Autodesk Inventor part; units mm, degrees
(part 3 of 3)
sketch "Sketch11" plane through (0, 0, 6.35) normal (0, 0, 1) x (1, 0, 0)
  line L0 (-44.1315, -133.8713) -> (-53.8141, -133.1794)
  arc A0 (-51.8719, -136.3964) -> (-74.636, -135.0027) centre (-63.5956, -141.2796) ccw projected
  line L1 (-36.4798, -134.4181) -> (-44.1315, -133.8713) projected
  arc A1 (-79.0465, -94.081) -> (-76.0542, -98.0205) centre (-69.1827, -89.6949) ccw projected
  line L2 (-76.0542, -98.0205) -> (-35.3561, -131.6103) projected
  arc A2 (-36.4798, -134.4181) -> (-35.3561, -131.6103) centre (-36.3666, -132.8347) ccw projected
  line L3 (-36.4798, -134.4181) -> (-44.1315, -133.8713) projected
  arc A3 (-44.1315, -133.8713) -> (-51.8719, -136.3964) centre (-44.901, -144.6389) ccw projected
  arc A4 (-51.8719, -136.3964) -> (-74.636, -135.0027) centre (-63.5956, -141.2796) ccw projected
  arc A5 (-85.5845, -139.4581) -> (-93.4453, -121.7039) centre (-97.0428, -133.914) ccw projected
  line L4 (-93.4453, -121.7039) -> (-88.3661, -96.7346) projected
  arc A6 (-88.3661, -96.7346) -> (-79.0465, -94.081) centre (-86.9165, -84.1335) ccw projected
  arc A7 (-88.6509, -203.8227) -> (-105.452, -206.2132) centre (-93.2079, -232.032) ccw projected
  arc A8 (-109.9237, -202.7115) -> (-105.452, -206.2132) centre (-106.8124, -203.3444) ccw projected
  line L5 (-109.9237, -202.7115) -> (-109.1471, -198.8936) projected
  arc A9 (-106.259, -196.3593) -> (-109.1471, -198.8936) centre (-106.0358, -199.5265) ccw projected
  arc A10 (-106.259, -196.3593) -> (-98.2138, -192.7133) centre (-107.1516, -183.6907) ccw projected
  arc A11 (-94.937, -191.9699) -> (-98.2138, -192.7133) centre (-95.9794, -194.9689) ccw projected
  line L6 (-94.937, -191.9699) -> (-86.0461, -195.0603) projected
  arc A12 (-84.1423, -199.2428) -> (-86.0461, -195.0603) centre (-87.0885, -198.0593) ccw projected
  line L7 (-84.1423, -199.2428) -> (-85.1984, -201.8718) projected
  arc A13 (-88.6509, -203.8227) -> (-85.1984, -201.8718) centre (-88.1445, -200.6883) ccw projected
  arc A14 (-28.8339, -52.5673) -> (-24.5425, -50.8749) centre (-27.4887, -49.6914) ccw projected
  line L8 (-28.8339, -52.5673) -> (-62.2456, -36.9383) projected
  arc A15 (-64.0748, -34.1198) -> (-62.2456, -36.9383) centre (-60.9004, -34.0624) ccw projected
  arc A16 (-64.0748, -34.1198) -> (-69.5395, -23.9103) centre (-76.7728, -34.3492) ccw projected
  arc A17 (-70.5556, -19.8503) -> (-69.5395, -23.9103) centre (-67.7312, -21.3006) ccw projected
  arc A18 (-64.7921, -10.8231) -> (-70.5556, -19.8503) centre (-19.7163, -45.9555) ccw projected
  line L9 (-64.7921, -10.8231) -> (-52.5861, 4.8375) projected
  arc A19 (-46.9122, 2.703) -> (-52.5861, 4.8375) centre (-50.0819, 2.8857) ccw projected
  arc A20 (-46.9122, 2.703) -> (-23.4164, -40.7398) centre (0, 0) ccw projected
  arc A21 (-22.0524, -44.676) -> (-23.4164, -40.7398) centre (-24.9986, -43.4925) ccw projected
  line L10 (-22.0524, -44.676) -> (-24.5425, -50.8749) projected
  arc A22 (-88.5389, -146.9454) -> (-92.3649, -145.7242) centre (-91.1997, -148.6777) ccw projected
  line L11 (-88.5389, -146.9454) -> (-60.6625, -189.7642) projected
  arc A23 (-61.0938, -193.7571) -> (-60.6625, -189.7642) centre (-63.3233, -191.4965) ccw projected
  arc A24 (-61.0938, -193.7571) -> (-61.1139, -193.7769) centre (-52.1761, -202.7994) ccw projected
  arc A25 (-64.3907, -194.5202) -> (-61.1139, -193.7769) centre (-63.3483, -191.5212) ccw projected
  line L12 (-64.3907, -194.5202) -> (-92.4352, -184.7723) projected
  arc A26 (-94.5445, -182.1568) -> (-92.4352, -184.7723) centre (-91.3928, -181.7733) ccw projected
  arc A27 (-94.5445, -182.1568) -> (-101.3806, -172.3776) centre (-107.1516, -183.6907) ccw projected
  arc A28 (-103.0492, -168.9165) -> (-101.3806, -172.3776) centre (-99.9379, -169.5493) ccw projected
  line L13 (-103.0492, -168.9165) -> (-99.0208, -149.1131) projected
  arc A29 (-96.1327, -146.5788) -> (-99.0208, -149.1131) centre (-95.9095, -149.746) ccw projected
  arc A30 (-96.1327, -146.5788) -> (-92.3649, -145.7242) centre (-97.0253, -133.9102) ccw projected
  arc A31 (-17.7613, -54.4362) -> (-16.1603, -58.4956) centre (-14.8151, -55.6197) ccw projected
  line L14 (-17.7613, -54.4362) -> (-14.9815, -47.5164) projected
  arc A32 (-11.2736, -45.6176) -> (-14.9815, -47.5164) centre (-12.0354, -48.6999) ccw projected
  arc A33 (-11.2736, -45.6176) -> (22.335, -41.3425) centre (0, 0) ccw projected
  arc A34 (26.6735, -45.5766) -> (22.335, -41.3425) centre (23.8442, -44.136) ccw projected
  line L15 (26.6735, -45.5766) -> (18.348, -61.9272) projected
  arc A35 (14.8879, -63.5983) -> (18.348, -61.9272) centre (15.5186, -60.4865) ccw projected
  arc A36 (14.8879, -63.5983) -> (4.4026, -66.1514) centre (12.3652, -76.0452) ccw projected
  arc A37 (1.0666, -66.5539) -> (4.4026, -66.1514) centre (2.4119, -63.6779) ccw projected
  line L16 (1.0666, -66.5539) -> (-16.1603, -58.4956) projected
  arc A38 (-75.9857, -77.6344) -> (-81.1281, -72.8166) centre (-86.899, -84.1297) ccw projected
  arc A39 (-82.7967, -69.3554) -> (-81.1281, -72.8166) centre (-79.6854, -69.9883) ccw projected
  line L17 (-82.7967, -69.3554) -> (-78.7683, -49.5521) projected
  arc A40 (-75.8802, -47.0178) -> (-78.7683, -49.5521) centre (-75.657, -50.185) ccw projected
  arc A41 (-75.8802, -47.0178) -> (-68.8102, -44.243) centre (-76.7728, -34.3492) ccw projected
  arc A42 (-65.4743, -43.8405) -> (-68.8102, -44.243) centre (-66.8195, -46.7164) ccw projected
  line L18 (-65.4743, -43.8405) -> (-13.0907, -68.3439) projected
  arc A43 (-14.1782, -74.3844) -> (-13.0907, -68.3439) centre (-14.436, -71.2199) ccw projected
  line L19 (-14.1782, -74.3844) -> (-72.9996, -79.1751) projected
  arc A44 (-75.9857, -77.6344) -> (-72.9996, -79.1751) centre (-73.2574, -76.0105) ccw projected
  arc A45 (1.4518, -82.5405) -> (3.7832, -85.4068) centre (12.3652, -76.0452) ccw projected
  arc A46 (4.4671, -89.1879) -> (3.7832, -85.4068) centre (1.6378, -87.7473) ccw projected
  line L20 (4.4671, -89.1879) -> (-13.923, -125.3043) projected
  arc A47 (-17.3829, -126.9753) -> (-13.923, -125.3043) centre (-16.7523, -123.8636) ccw projected
  arc A48 (-17.3829, -126.9753) -> (-25.1442, -127.8531) centre (-19.9055, -139.4223) ccw projected
  arc A49 (-28.4749, -127.4095) -> (-25.1442, -127.8531) centre (-26.4539, -124.9608) ccw projected
  line L21 (-28.4749, -127.4095) -> (-71.2037, -92.1436) projected
  arc A50 (-69.4404, -86.5304) -> (-71.2037, -92.1436) centre (-69.1827, -89.6949) ccw projected
  line L22 (-69.4404, -86.5304) -> (-1.5342, -80.9998) projected
  arc A51 (1.4518, -82.5405) -> (-1.5342, -80.9998) centre (-1.2765, -84.1643) ccw projected
  arc A52 (-64.7831, -204.3333) -> (-60.7584, -212.1608) centre (-52.1761, -202.7994) ccw projected
  arc A53 (-60.0746, -215.9418) -> (-60.7584, -212.1608) centre (-62.9039, -214.5011) ccw projected
  line L23 (-60.0746, -215.9418) -> (-61.8773, -219.482) projected
  arc A54 (-67.5567, -219.4404) -> (-61.8773, -219.482) centre (-64.7066, -218.0413) ccw projected
  arc A55 (-67.5567, -219.4404) -> (-76.984, -208.5093) centre (-93.2079, -232.032) ccw projected
  arc A56 (-78.1275, -204.7122) -> (-76.984, -208.5093) centre (-75.1814, -205.8957) ccw projected
  line L24 (-78.1275, -204.7122) -> (-76.8242, -201.4676) projected
  arc A57 (-72.8356, -199.6521) -> (-76.8242, -201.4676) centre (-73.878, -202.6511) ccw projected
  line L25 (-72.8356, -199.6521) -> (-66.8925, -201.7178) projected
  arc A58 (-64.7831, -204.3333) -> (-66.8925, -201.7178) centre (-67.9349, -204.7168) ccw projected
  circle A59 centre (-19.9058, -139.422) radius 5.588 projected
  circle A60 centre (-107.169, -183.6945) radius 5.588 projected
  circle A61 centre (-86.9165, -84.1335) radius 5.588 projected
  circle A62 centre (-56.5448, -157.7983) radius 6.731 projected
  line L26 (-98.521, -236.7409) -> (-93.7871, -224.9561) projected
  arc A63 (-87.8947, -227.3231) -> (-93.7871, -224.9561) centre (-90.8409, -226.1396) ccw projected
  line L27 (-87.8947, -227.3231) -> (-92.6287, -239.1078) projected
  arc A64 (-98.521, -236.7409) -> (-92.6287, -239.1078) centre (-95.5749, -237.9244) ccw projected
  circle A65 centre (0, 0) radius 13.4938 projected
  arc A66 (56.5866, -28.8133) -> (-50.0843, 39.0361) centre (0, 0) ccw projected
  line L28 (-50.0843, 39.0361) -> (-79.8174, 0.8878) projected
  arc A67 (-79.8174, 0.8878) -> (-94.387, -30.7661) centre (-19.7163, -45.9555) ccw projected
  line L29 (-94.387, -30.7661) -> (-133.6545, -223.8044) projected
  arc A68 (-133.6545, -223.8044) -> (-56.4266, -250.7606) centre (-93.2079, -232.032) ccw projected
  line L30 (-56.4266, -250.7606) -> (56.5866, -28.8133) projected
  circle A69 centre (-63.5956, -141.2796) radius 6.731 projected
  arc A70 (-11.6072, -28.8689) -> (-9.2419, -22.976) centre (-10.4066, -25.9296) ccw projected
  arc A71 (-9.2419, -22.976) -> (-11.6072, -28.8689) centre (-10.4425, -25.9152) ccw projected
  arc A72 (26.3454, 16.5542) -> (20.9946, 13.1351) centre (23.6593, 14.8615) ccw projected
  arc A73 (20.9946, 13.1351) -> (26.3454, 16.5542) centre (23.6807, 14.8279) ccw projected
  arc A74 (23.8979, -19.9247) -> (18.9666, -15.9242) centre (21.4446, -17.9092) ccw projected
  arc A75 (18.9666, -15.9242) -> (23.8979, -19.9247) centre (21.4199, -17.9397) ccw projected
  arc A76 (-7.5477, 30.1857) -> (-6.0599, 24.0126) centre (-6.8231, 27.0945) ccw projected
  arc A77 (-6.0599, 24.0126) -> (-7.5477, 30.1857) centre (-6.7844, 27.1038) ccw projected
  arc A78 (-31.0394, 2.1661) -> (-24.7113, 1.6412) centre (-27.877, 1.8842) ccw projected
  arc A79 (-24.7113, 1.6412) -> (-31.0394, 2.1661) centre (-27.8737, 1.9232) ccw projected
  circle A80 centre (-76.7902, -34.353) radius 5.588 projected
  circle A81 centre (-97.0428, -133.914) radius 5.588 projected
  circle A82 centre (12.3653, -76.0452) radius 5.588 projected
  circle A83 centre (-52.177, -202.7989) radius 5.588 projected
  point P0 (0, 0)
  point P1 (-51.8719, -136.3964)
  point P2 (-44.1315, -133.8713)
  constraints: 2 end point, 1 collinear, 1 point on circle, 1 other
extrude "Extrusion11" add sketch "Sketch11" against normal blind 6.35 contours A3 A0 L0
sketch "Sketch12" plane through (0, 0, 6.35) normal (0, 0, 1) x (1, 0, 0)
  line L0 (-36.4798, -134.4181) -> (-53.8141, -133.1794) projected
  line L1 (-53.8141, -133.1794) -> (-84.6576, -130.9752)
  arc A0 (-85.5845, -139.4581) -> (-93.4453, -121.7039) centre (-97.0428, -133.914) ccw projected
  arc A1 (-79.0465, -94.081) -> (-76.0542, -98.0205) centre (-69.1827, -89.6949) ccw projected
  line L2 (-76.0542, -98.0205) -> (-35.3561, -131.6103) projected
  arc A2 (-36.4798, -134.4181) -> (-35.3561, -131.6103) centre (-36.3666, -132.8347) ccw projected
  line L3 (-36.4798, -134.4181) -> (-53.8141, -133.1794) projected
  arc A3 (-53.8141, -133.1794) -> (-74.636, -135.0027) centre (-63.5956, -141.2796) ccw projected
  spline S0 degree 4 poles (-74.636, -135.0027) (-76.6708, -138.5198) (-78.5316, -143.7344) (-82.756, -141.1808) (-85.5845, -139.4581) knots 0 0 0 0 0 1 1 1 1 1 projected
  arc A4 (-85.5845, -139.4581) -> (-93.4453, -121.7039) centre (-97.0428, -133.914) ccw projected
  line L4 (-93.4453, -121.7039) -> (-88.3661, -96.7346) projected
  arc A5 (-88.3661, -96.7346) -> (-79.0465, -94.081) centre (-86.9165, -84.1335) ccw projected
  arc A6 (-88.6509, -203.8227) -> (-105.452, -206.2132) centre (-93.2079, -232.032) ccw projected
  arc A7 (-109.9237, -202.7115) -> (-105.452, -206.2132) centre (-106.8124, -203.3444) ccw projected
  line L5 (-109.9237, -202.7115) -> (-109.1471, -198.8936) projected
  arc A8 (-106.259, -196.3593) -> (-109.1471, -198.8936) centre (-106.0358, -199.5265) ccw projected
  arc A9 (-106.259, -196.3593) -> (-98.2138, -192.7133) centre (-107.1516, -183.6907) ccw projected
  arc A10 (-94.937, -191.9699) -> (-98.2138, -192.7133) centre (-95.9794, -194.9689) ccw projected
  line L6 (-94.937, -191.9699) -> (-86.0461, -195.0603) projected
  arc A11 (-84.1423, -199.2428) -> (-86.0461, -195.0603) centre (-87.0885, -198.0593) ccw projected
  line L7 (-84.1423, -199.2428) -> (-85.1984, -201.8718) projected
  arc A12 (-88.6509, -203.8227) -> (-85.1984, -201.8718) centre (-88.1445, -200.6883) ccw projected
  arc A13 (-28.8339, -52.5673) -> (-24.5425, -50.8749) centre (-27.4887, -49.6914) ccw projected
  line L8 (-28.8339, -52.5673) -> (-62.2456, -36.9383) projected
  arc A14 (-64.0748, -34.1198) -> (-62.2456, -36.9383) centre (-60.9004, -34.0624) ccw projected
  arc A15 (-64.0748, -34.1198) -> (-69.5395, -23.9103) centre (-76.7728, -34.3492) ccw projected
  arc A16 (-70.5556, -19.8503) -> (-69.5395, -23.9103) centre (-67.7312, -21.3006) ccw projected
  arc A17 (-64.7921, -10.8231) -> (-70.5556, -19.8503) centre (-19.7163, -45.9555) ccw projected
  line L9 (-64.7921, -10.8231) -> (-52.5861, 4.8375) projected
  arc A18 (-46.9122, 2.703) -> (-52.5861, 4.8375) centre (-50.0819, 2.8857) ccw projected
  arc A19 (-46.9122, 2.703) -> (-23.4164, -40.7398) centre (0, 0) ccw projected
  arc A20 (-22.0524, -44.676) -> (-23.4164, -40.7398) centre (-24.9986, -43.4925) ccw projected
  line L10 (-22.0524, -44.676) -> (-24.5425, -50.8749) projected
  arc A21 (-88.5389, -146.9454) -> (-92.3649, -145.7242) centre (-91.1997, -148.6777) ccw projected
  line L11 (-88.5389, -146.9454) -> (-60.6625, -189.7642) projected
  arc A22 (-61.0938, -193.7571) -> (-60.6625, -189.7642) centre (-63.3233, -191.4965) ccw projected
  arc A23 (-61.0938, -193.7571) -> (-61.1139, -193.7769) centre (-52.1761, -202.7994) ccw projected
  arc A24 (-64.3907, -194.5202) -> (-61.1139, -193.7769) centre (-63.3483, -191.5212) ccw projected
  line L12 (-64.3907, -194.5202) -> (-92.4352, -184.7723) projected
  arc A25 (-94.5445, -182.1568) -> (-92.4352, -184.7723) centre (-91.3928, -181.7733) ccw projected
  arc A26 (-94.5445, -182.1568) -> (-101.3806, -172.3776) centre (-107.1516, -183.6907) ccw projected
  arc A27 (-103.0492, -168.9165) -> (-101.3806, -172.3776) centre (-99.9379, -169.5493) ccw projected
  line L13 (-103.0492, -168.9165) -> (-99.0208, -149.1131) projected
  arc A28 (-96.1327, -146.5788) -> (-99.0208, -149.1131) centre (-95.9095, -149.746) ccw projected
  arc A29 (-96.1327, -146.5788) -> (-92.3649, -145.7242) centre (-97.0253, -133.9102) ccw projected
  arc A30 (-17.7613, -54.4362) -> (-16.1603, -58.4956) centre (-14.8151, -55.6197) ccw projected
  line L14 (-17.7613, -54.4362) -> (-14.9815, -47.5164) projected
  arc A31 (-11.2736, -45.6176) -> (-14.9815, -47.5164) centre (-12.0354, -48.6999) ccw projected
  arc A32 (-11.2736, -45.6176) -> (22.335, -41.3425) centre (0, 0) ccw projected
  arc A33 (26.6735, -45.5766) -> (22.335, -41.3425) centre (23.8442, -44.136) ccw projected
  line L15 (26.6735, -45.5766) -> (18.348, -61.9272) projected
  arc A34 (14.8879, -63.5983) -> (18.348, -61.9272) centre (15.5186, -60.4865) ccw projected
  arc A35 (14.8879, -63.5983) -> (4.4026, -66.1514) centre (12.3652, -76.0452) ccw projected
  arc A36 (1.0666, -66.5539) -> (4.4026, -66.1514) centre (2.4119, -63.6779) ccw projected
  line L16 (1.0666, -66.5539) -> (-16.1603, -58.4956) projected
  arc A37 (-75.9857, -77.6344) -> (-81.1281, -72.8166) centre (-86.899, -84.1297) ccw projected
  arc A38 (-82.7967, -69.3554) -> (-81.1281, -72.8166) centre (-79.6854, -69.9883) ccw projected
  line L17 (-82.7967, -69.3554) -> (-78.7683, -49.5521) projected
  arc A39 (-75.8802, -47.0178) -> (-78.7683, -49.5521) centre (-75.657, -50.185) ccw projected
  arc A40 (-75.8802, -47.0178) -> (-68.8102, -44.243) centre (-76.7728, -34.3492) ccw projected
  arc A41 (-65.4743, -43.8405) -> (-68.8102, -44.243) centre (-66.8195, -46.7164) ccw projected
  line L18 (-65.4743, -43.8405) -> (-13.0907, -68.3439) projected
  arc A42 (-14.1782, -74.3844) -> (-13.0907, -68.3439) centre (-14.436, -71.2199) ccw projected
  line L19 (-14.1782, -74.3844) -> (-72.9996, -79.1751) projected
  arc A43 (-75.9857, -77.6344) -> (-72.9996, -79.1751) centre (-73.2574, -76.0105) ccw projected
  arc A44 (1.4518, -82.5405) -> (3.7832, -85.4068) centre (12.3652, -76.0452) ccw projected
  arc A45 (4.4671, -89.1879) -> (3.7832, -85.4068) centre (1.6378, -87.7473) ccw projected
  line L20 (4.4671, -89.1879) -> (-13.923, -125.3043) projected
  arc A46 (-17.3829, -126.9753) -> (-13.923, -125.3043) centre (-16.7523, -123.8636) ccw projected
  arc A47 (-17.3829, -126.9753) -> (-25.1442, -127.8531) centre (-19.9055, -139.4223) ccw projected
  arc A48 (-28.4749, -127.4095) -> (-25.1442, -127.8531) centre (-26.4539, -124.9608) ccw projected
  line L21 (-28.4749, -127.4095) -> (-71.2037, -92.1436) projected
  arc A49 (-69.4404, -86.5304) -> (-71.2037, -92.1436) centre (-69.1827, -89.6949) ccw projected
  line L22 (-69.4404, -86.5304) -> (-1.5342, -80.9998) projected
  arc A50 (1.4518, -82.5405) -> (-1.5342, -80.9998) centre (-1.2765, -84.1643) ccw projected
  arc A51 (-64.7831, -204.3333) -> (-60.7584, -212.1608) centre (-52.1761, -202.7994) ccw projected
  arc A52 (-60.0746, -215.9418) -> (-60.7584, -212.1608) centre (-62.9039, -214.5011) ccw projected
  line L23 (-60.0746, -215.9418) -> (-61.8773, -219.482) projected
  arc A53 (-67.5567, -219.4404) -> (-61.8773, -219.482) centre (-64.7066, -218.0413) ccw projected
  arc A54 (-67.5567, -219.4404) -> (-76.984, -208.5093) centre (-93.2079, -232.032) ccw projected
  arc A55 (-78.1275, -204.7122) -> (-76.984, -208.5093) centre (-75.1814, -205.8957) ccw projected
  line L24 (-78.1275, -204.7122) -> (-76.8242, -201.4676) projected
  arc A56 (-72.8356, -199.6521) -> (-76.8242, -201.4676) centre (-73.878, -202.6511) ccw projected
  line L25 (-72.8356, -199.6521) -> (-66.8925, -201.7178) projected
  arc A57 (-64.7831, -204.3333) -> (-66.8925, -201.7178) centre (-67.9349, -204.7168) ccw projected
  circle A58 centre (-19.9058, -139.422) radius 5.588 projected
  circle A59 centre (-107.169, -183.6945) radius 5.588 projected
  circle A60 centre (-86.9165, -84.1335) radius 5.588 projected
  circle A61 centre (-56.5448, -157.7983) radius 6.731 projected
  line L26 (-98.521, -236.7409) -> (-93.7871, -224.9561) projected
  arc A62 (-87.8947, -227.3231) -> (-93.7871, -224.9561) centre (-90.8409, -226.1396) ccw projected
  line L27 (-87.8947, -227.3231) -> (-92.6287, -239.1078) projected
  arc A63 (-98.521, -236.7409) -> (-92.6287, -239.1078) centre (-95.5749, -237.9244) ccw projected
  circle A64 centre (0, 0) radius 13.4938 projected
  arc A65 (56.5866, -28.8133) -> (-50.0843, 39.0361) centre (0, 0) ccw projected
  line L28 (-50.0843, 39.0361) -> (-79.8174, 0.8878) projected
  arc A66 (-79.8174, 0.8878) -> (-94.387, -30.7661) centre (-19.7163, -45.9555) ccw projected
  line L29 (-94.387, -30.7661) -> (-133.6545, -223.8044) projected
  arc A67 (-133.6545, -223.8044) -> (-56.4266, -250.7606) centre (-93.2079, -232.032) ccw projected
  line L30 (-56.4266, -250.7606) -> (56.5866, -28.8133) projected
  circle A68 centre (-63.5956, -141.2796) radius 6.731 projected
  arc A69 (-11.6072, -28.8689) -> (-9.2419, -22.976) centre (-10.4066, -25.9296) ccw projected
  arc A70 (-9.2419, -22.976) -> (-11.6072, -28.8689) centre (-10.4425, -25.9152) ccw projected
  arc A71 (26.3454, 16.5542) -> (20.9946, 13.1351) centre (23.6593, 14.8615) ccw projected
  arc A72 (20.9946, 13.1351) -> (26.3454, 16.5542) centre (23.6807, 14.8279) ccw projected
  arc A73 (23.8979, -19.9247) -> (18.9666, -15.9242) centre (21.4446, -17.9092) ccw projected
  arc A74 (18.9666, -15.9242) -> (23.8979, -19.9247) centre (21.4199, -17.9397) ccw projected
  arc A75 (-7.5477, 30.1857) -> (-6.0599, 24.0126) centre (-6.8231, 27.0945) ccw projected
  arc A76 (-6.0599, 24.0126) -> (-7.5477, 30.1857) centre (-6.7844, 27.1038) ccw projected
  arc A77 (-31.0394, 2.1661) -> (-24.7113, 1.6412) centre (-27.877, 1.8842) ccw projected
  arc A78 (-24.7113, 1.6412) -> (-31.0394, 2.1661) centre (-27.8737, 1.9232) ccw projected
  circle A79 centre (-76.7902, -34.353) radius 5.588 projected
  circle A80 centre (-97.0428, -133.914) radius 5.588 projected
  circle A81 centre (12.3653, -76.0452) radius 5.588 projected
  circle A82 centre (-52.177, -202.7989) radius 5.588 projected
  point P0 (0, 0)
  point P1 (-85.5845, -139.4581)
  point P2 (-72.1258, -131.8708)
  constraints: 2 end point, 1 collinear, 1 point on circle, 1 other
extrude "Extrusion12" add sketch "Sketch12" against normal blind 6.35 contours A3 S0 A0 L1
fillet "Fillet2" radius 3.175 6 edges at (-93.4453, -121.7039, 3.175) (-84.6576, -130.9752, 3.175) (-79.0465, -94.081, 3.175) (-88.3661, -96.7346, 3.175) (-72.1258, -131.8708, 3.175) (-53.8141, -133.1794, 3.175)
sketch "Sketch13" plane through (0, 0, 6.35) normal (0, 0, 1) x (1, 0, 0)
  circle A0 centre (-97.0428, -133.914) radius 2.413 projected
  circle A1 centre (-52.177, -202.7989) radius 2.413 projected
  line L0 (-97.0428, -133.914) -> (-52.177, -202.7989)
  line L1 (-100.2361, -135.9922) -> (-55.377, -204.8667)
  arc A2 (-77.6001, -96.4537) -> (-76.0542, -98.0205) centre (-69.1827, -89.6949) ccw projected
  line L2 (-76.0542, -98.0205) -> (-35.3561, -131.6103) projected
  arc A3 (-36.4798, -134.4181) -> (-35.3561, -131.6103) centre (-36.3666, -132.8347) ccw projected
  line L3 (-36.4798, -134.4181) -> (-52.5481, -133.2699) projected
  arc A4 (-54.5766, -132.3383) -> (-52.5481, -133.2699) centre (-52.3218, -130.1029) ccw projected
  arc A5 (-54.5766, -132.3383) -> (-71.2515, -131.1466) centre (-63.5956, -141.2796) ccw projected
  arc A6 (-73.3918, -131.7803) -> (-71.2515, -131.1466) centre (-73.1655, -128.6134) ccw projected
  line L4 (-73.3918, -131.7803) -> (-82.5212, -131.1279) projected
  arc A7 (-85.2391, -129.1494) -> (-82.5212, -131.1279) centre (-82.2949, -127.961) ccw projected
  arc A8 (-85.2391, -129.1494) -> (-91.2523, -122.5783) centre (-97.0428, -133.914) ccw projected
  arc A9 (-92.9193, -119.1179) -> (-91.2523, -122.5783) centre (-89.808, -119.7508) ccw projected
  line L5 (-92.9193, -119.1179) -> (-88.8918, -99.3191) projected
  arc A10 (-86.0079, -96.7851) -> (-88.8918, -99.3191) centre (-85.7805, -99.952) ccw projected
  arc A11 (-86.0079, -96.7851) -> (-81.4453, -95.5771) centre (-86.9165, -84.1335) ccw projected
  arc A12 (-77.6001, -96.4537) -> (-81.4453, -95.5771) centre (-80.0758, -98.4415) ccw projected
  arc A13 (-88.6509, -203.8227) -> (-105.452, -206.2132) centre (-93.2079, -232.032) ccw projected
  arc A14 (-109.9237, -202.7115) -> (-105.452, -206.2132) centre (-106.8124, -203.3444) ccw projected
  line L6 (-109.9237, -202.7115) -> (-109.1471, -198.8936) projected
  arc A15 (-106.259, -196.3593) -> (-109.1471, -198.8936) centre (-106.0358, -199.5265) ccw projected
  arc A16 (-106.259, -196.3593) -> (-98.2138, -192.7133) centre (-107.1516, -183.6907) ccw projected
  arc A17 (-94.937, -191.9699) -> (-98.2138, -192.7133) centre (-95.9794, -194.9689) ccw projected
  line L7 (-94.937, -191.9699) -> (-86.0461, -195.0603) projected
  arc A18 (-84.1423, -199.2428) -> (-86.0461, -195.0603) centre (-87.0885, -198.0593) ccw projected
  line L8 (-84.1423, -199.2428) -> (-85.1984, -201.8718) projected
  arc A19 (-88.6509, -203.8227) -> (-85.1984, -201.8718) centre (-88.1445, -200.6883) ccw projected
  arc A20 (-28.8339, -52.5673) -> (-24.5425, -50.8749) centre (-27.4887, -49.6914) ccw projected
  line L9 (-28.8339, -52.5673) -> (-62.2456, -36.9383) projected
  arc A21 (-64.0748, -34.1198) -> (-62.2456, -36.9383) centre (-60.9004, -34.0624) ccw projected
  arc A22 (-64.0748, -34.1198) -> (-69.5395, -23.9103) centre (-76.7728, -34.3492) ccw projected
  arc A23 (-70.5556, -19.8503) -> (-69.5395, -23.9103) centre (-67.7312, -21.3006) ccw projected
  arc A24 (-64.7921, -10.8231) -> (-70.5556, -19.8503) centre (-19.7163, -45.9555) ccw projected
  line L10 (-64.7921, -10.8231) -> (-52.5861, 4.8375) projected
  arc A25 (-46.9122, 2.703) -> (-52.5861, 4.8375) centre (-50.0819, 2.8857) ccw projected
  arc A26 (-46.9122, 2.703) -> (-23.4164, -40.7398) centre (0, 0) ccw projected
  arc A27 (-22.0524, -44.676) -> (-23.4164, -40.7398) centre (-24.9986, -43.4925) ccw projected
  line L11 (-22.0524, -44.676) -> (-24.5425, -50.8749) projected
  arc A28 (-88.5389, -146.9454) -> (-92.3649, -145.7242) centre (-91.1997, -148.6777) ccw projected
  line L12 (-88.5389, -146.9454) -> (-60.6625, -189.7642) projected
  arc A29 (-61.0938, -193.7571) -> (-60.6625, -189.7642) centre (-63.3233, -191.4965) ccw projected
  arc A30 (-61.0938, -193.7571) -> (-61.1139, -193.7769) centre (-52.1761, -202.7994) ccw projected
  arc A31 (-64.3907, -194.5202) -> (-61.1139, -193.7769) centre (-63.3483, -191.5212) ccw projected
  line L13 (-64.3907, -194.5202) -> (-92.4352, -184.7723) projected
  arc A32 (-94.5445, -182.1568) -> (-92.4352, -184.7723) centre (-91.3928, -181.7733) ccw projected
  arc A33 (-94.5445, -182.1568) -> (-101.3806, -172.3776) centre (-107.1516, -183.6907) ccw projected
  arc A34 (-103.0492, -168.9165) -> (-101.3806, -172.3776) centre (-99.9379, -169.5493) ccw projected
  line L14 (-103.0492, -168.9165) -> (-99.0208, -149.1131) projected
  arc A35 (-96.1327, -146.5788) -> (-99.0208, -149.1131) centre (-95.9095, -149.746) ccw projected
  arc A36 (-96.1327, -146.5788) -> (-92.3649, -145.7242) centre (-97.0253, -133.9102) ccw projected
  arc A37 (-17.7613, -54.4362) -> (-16.1603, -58.4956) centre (-14.8151, -55.6197) ccw projected
  line L15 (-17.7613, -54.4362) -> (-14.9815, -47.5164) projected
  arc A38 (-11.2736, -45.6176) -> (-14.9815, -47.5164) centre (-12.0354, -48.6999) ccw projected
  arc A39 (-11.2736, -45.6176) -> (22.335, -41.3425) centre (0, 0) ccw projected
  arc A40 (26.6735, -45.5766) -> (22.335, -41.3425) centre (23.8442, -44.136) ccw projected
  line L16 (26.6735, -45.5766) -> (18.348, -61.9272) projected
  arc A41 (14.8879, -63.5983) -> (18.348, -61.9272) centre (15.5186, -60.4865) ccw projected
  arc A42 (14.8879, -63.5983) -> (4.4026, -66.1514) centre (12.3652, -76.0452) ccw projected
  arc A43 (1.0666, -66.5539) -> (4.4026, -66.1514) centre (2.4119, -63.6779) ccw projected
  line L17 (1.0666, -66.5539) -> (-16.1603, -58.4956) projected
  arc A44 (-75.9857, -77.6344) -> (-81.1281, -72.8166) centre (-86.899, -84.1297) ccw projected
  arc A45 (-82.7967, -69.3554) -> (-81.1281, -72.8166) centre (-79.6854, -69.9883) ccw projected
  line L18 (-82.7967, -69.3554) -> (-78.7683, -49.5521) projected
  arc A46 (-75.8802, -47.0178) -> (-78.7683, -49.5521) centre (-75.657, -50.185) ccw projected
  arc A47 (-75.8802, -47.0178) -> (-68.8102, -44.243) centre (-76.7728, -34.3492) ccw projected
  arc A48 (-65.4743, -43.8405) -> (-68.8102, -44.243) centre (-66.8195, -46.7164) ccw projected
  line L19 (-65.4743, -43.8405) -> (-13.0907, -68.3439) projected
  arc A49 (-14.1782, -74.3844) -> (-13.0907, -68.3439) centre (-14.436, -71.2199) ccw projected
  line L20 (-14.1782, -74.3844) -> (-72.9996, -79.1751) projected
  arc A50 (-75.9857, -77.6344) -> (-72.9996, -79.1751) centre (-73.2574, -76.0105) ccw projected
  arc A51 (1.4518, -82.5405) -> (3.7832, -85.4068) centre (12.3652, -76.0452) ccw projected
  arc A52 (4.4671, -89.1879) -> (3.7832, -85.4068) centre (1.6378, -87.7473) ccw projected
  line L21 (4.4671, -89.1879) -> (-13.923, -125.3043) projected
  arc A53 (-17.3829, -126.9753) -> (-13.923, -125.3043) centre (-16.7523, -123.8636) ccw projected
  arc A54 (-17.3829, -126.9753) -> (-25.1442, -127.8531) centre (-19.9055, -139.4223) ccw projected
  arc A55 (-28.4749, -127.4095) -> (-25.1442, -127.8531) centre (-26.4539, -124.9608) ccw projected
  line L22 (-28.4749, -127.4095) -> (-71.2037, -92.1436) projected
  arc A56 (-69.4404, -86.5304) -> (-71.2037, -92.1436) centre (-69.1827, -89.6949) ccw projected
  line L23 (-69.4404, -86.5304) -> (-1.5342, -80.9998) projected
  arc A57 (1.4518, -82.5405) -> (-1.5342, -80.9998) centre (-1.2765, -84.1643) ccw projected
  arc A58 (-64.7831, -204.3333) -> (-60.7584, -212.1608) centre (-52.1761, -202.7994) ccw projected
  arc A59 (-60.0746, -215.9418) -> (-60.7584, -212.1608) centre (-62.9039, -214.5011) ccw projected
  line L24 (-60.0746, -215.9418) -> (-61.8773, -219.482) projected
  arc A60 (-67.5567, -219.4404) -> (-61.8773, -219.482) centre (-64.7066, -218.0413) ccw projected
  arc A61 (-67.5567, -219.4404) -> (-76.984, -208.5093) centre (-93.2079, -232.032) ccw projected
  arc A62 (-78.1275, -204.7122) -> (-76.984, -208.5093) centre (-75.1814, -205.8957) ccw projected
  line L25 (-78.1275, -204.7122) -> (-76.8242, -201.4676) projected
  arc A63 (-72.8356, -199.6521) -> (-76.8242, -201.4676) centre (-73.878, -202.6511) ccw projected
  line L26 (-72.8356, -199.6521) -> (-66.8925, -201.7178) projected
  arc A64 (-64.7831, -204.3333) -> (-66.8925, -201.7178) centre (-67.9349, -204.7168) ccw projected
  circle A65 centre (-19.9058, -139.422) radius 5.588 projected
  circle A66 centre (-107.169, -183.6945) radius 5.588 projected
  circle A67 centre (-86.9165, -84.1335) radius 5.588 projected
  circle A68 centre (-56.5448, -157.7983) radius 6.731 projected
  line L27 (-98.521, -236.7409) -> (-93.7871, -224.9561) projected
  arc A69 (-87.8947, -227.3231) -> (-93.7871, -224.9561) centre (-90.8409, -226.1396) ccw projected
  line L28 (-87.8947, -227.3231) -> (-92.6287, -239.1078) projected
  arc A70 (-98.521, -236.7409) -> (-92.6287, -239.1078) centre (-95.5749, -237.9244) ccw projected
  circle A71 centre (0, 0) radius 13.4938 projected
  arc A72 (56.5866, -28.8133) -> (-50.0843, 39.0361) centre (0, 0) ccw projected
  line L29 (-50.0843, 39.0361) -> (-79.8174, 0.8878) projected
  arc A73 (-79.8174, 0.8878) -> (-94.387, -30.7661) centre (-19.7163, -45.9555) ccw projected
  line L30 (-94.387, -30.7661) -> (-133.6545, -223.8044) projected
  arc A74 (-133.6545, -223.8044) -> (-56.4266, -250.7606) centre (-93.2079, -232.032) ccw projected
  line L31 (-56.4266, -250.7606) -> (56.5866, -28.8133) projected
  circle A75 centre (-63.5956, -141.2796) radius 6.731 projected
  arc A76 (-11.6072, -28.8689) -> (-9.2419, -22.976) centre (-10.4066, -25.9296) ccw projected
  arc A77 (-9.2419, -22.976) -> (-11.6072, -28.8689) centre (-10.4425, -25.9152) ccw projected
  arc A78 (26.3454, 16.5542) -> (20.9946, 13.1351) centre (23.6593, 14.8615) ccw projected
  arc A79 (20.9946, 13.1351) -> (26.3454, 16.5542) centre (23.6807, 14.8279) ccw projected
  arc A80 (23.8979, -19.9247) -> (18.9666, -15.9242) centre (21.4446, -17.9092) ccw projected
  arc A81 (18.9666, -15.9242) -> (23.8979, -19.9247) centre (21.4199, -17.9397) ccw projected
  arc A82 (-7.5477, 30.1857) -> (-6.0599, 24.0126) centre (-6.8231, 27.0945) ccw projected
  arc A83 (-6.0599, 24.0126) -> (-7.5477, 30.1857) centre (-6.7844, 27.1038) ccw projected
  arc A84 (-31.0394, 2.1661) -> (-24.7113, 1.6412) centre (-27.877, 1.8842) ccw projected
  arc A85 (-24.7113, 1.6412) -> (-31.0394, 2.1661) centre (-27.8737, 1.9232) ccw projected
  circle A86 centre (-76.7902, -34.353) radius 5.588 projected
  circle A87 centre (-97.0428, -133.914) radius 5.588 projected
  circle A88 centre (12.3653, -76.0452) radius 5.588 projected
  circle A89 centre (-52.177, -202.7989) radius 5.588 projected
  point P0 (0, 0)
  point P1 (-93.6228, -146.1459)
  point P2 (-62.1533, -194.4628)
  dimension "d55" = 3.81
  constraints: 4 end point, 1 parallel
  measures "d55" distance between parallel lines of L0 L1
extrude "Extrusion13" add sketch "Sketch13" against normal blind 6.35 contours A28 L12 A29 L0 | L0 A29 A30 A31 L1 A36 A28
fillet "Fillet3" radius 3.175 2 edges at (-93.6228, -146.1459, 3.175) (-62.1533, -194.4628, 3.175)
sketch "Sketch14" plane through (0, 0, 6.35) normal (0, 0, 1) x (1, 0, 0)
  arc A0 (-82.2866, -251.3886) -> (-73.4026, -242.1166) centre (-93.2079, -232.032) ccw projected
  line L0 (-73.4026, -242.1166) -> (-72.5842, -240.5094) projected
  arc A1 (-72.5842, -240.5094) -> (-73.2785, -238.3744) centre (-73.9989, -239.7891) ccw projected
  line L1 (-73.2785, -238.3744) -> (-79.039, -235.4413) projected
  arc A2 (-79.039, -235.4413) -> (-81.2537, -236.3199) centre (-79.7594, -236.8559) ccw projected
  arc A3 (-82.9809, -239.5618) -> (-81.2537, -236.3199) centre (-93.2079, -232.032) ccw projected
  arc A4 (-86.1924, -246.4835) -> (-82.9809, -239.5618) centre (-95.5749, -237.9244) ccw projected
  arc A5 (-86.1924, -246.4835) -> (-82.2866, -251.3886) centre (-83.8468, -248.6233) ccw projected
  arc A6 (-107.2952, -233.0332) -> (-109.5924, -228.6991) centre (-110.2253, -231.8104) ccw projected
  line L2 (-109.5924, -228.6991) -> (-113.3713, -227.9304) projected
  arc A7 (-113.3713, -227.9304) -> (-115.2631, -229.2902) centre (-113.6877, -229.486) ccw projected
  arc A8 (-115.2631, -229.2902) -> (-114.4847, -238.4545) centre (-93.2079, -232.032) ccw projected
  arc A9 (-114.4847, -238.4545) -> (-108.2711, -237.6145) centre (-111.4451, -237.537) ccw projected
  arc A10 (-107.2952, -233.0332) -> (-108.2711, -237.6145) centre (-95.5749, -237.9244) ccw projected
  arc A11 (35.5169, -0.0989) -> (38.7459, 3.1685) centre (23.6807, 14.8279) ccw projected
  arc A12 (35.5169, -0.0989) -> (35.1939, -4.7799) centre (37.4896, -2.5866) ccw projected
  arc A13 (37.9436, -8.4597) -> (35.1939, -4.7799) centre (21.4199, -17.9397) ccw projected
  arc A14 (37.9436, -8.4597) -> (43.8282, -7.409) centre (40.6976, -6.8798) ccw projected
  arc A15 (43.8282, -7.409) -> (44.4304, 1.3195) centre (0, 0) ccw projected
  arc A16 (44.4304, 1.3195) -> (38.7459, 3.1685) centre (41.2568, 1.2252) ccw projected
  arc A17 (11.0693, 33.748) -> (8.9598, 37.8287) centre (-6.7844, 27.1038) ccw projected
  arc A18 (11.0693, 33.748) -> (15.4215, 31.9943) centre (14.045, 34.8554) ccw projected
  arc A19 (19.7709, 33.4723) -> (15.4215, 31.9943) centre (23.6807, 14.8279) ccw projected
  arc A20 (19.7709, 33.4723) -> (20.59, 39.3936) centre (19.1193, 36.5798) ccw projected
  arc A21 (20.59, 39.3936) -> (12.4749, 42.6636) centre (0, 0) ccw projected
  arc A22 (12.4749, 42.6636) -> (8.9598, 37.8287) centre (11.5838, 39.6162) ccw projected
  arc A23 (-31.1029, 31.7555) -> (-35.059, 27.3253) centre (0, 0) ccw projected
  line L3 (-35.059, 27.3253) -> (-36.7385, 25.1704) projected
  arc A24 (-36.7385, 25.1704) -> (-33.3257, 20.1764) centre (-34.2343, 23.2186) ccw projected
  arc A25 (-28.6757, 20.9563) -> (-33.3257, 20.1764) centre (-27.8737, 1.9232) ccw projected
  arc A26 (-28.6757, 20.9563) -> (-25.6629, 24.5535) centre (-28.8093, 24.1285) ccw projected
  arc A27 (-25.7245, 29.1468) -> (-25.6629, 24.5535) centre (-6.7844, 27.1038) ccw projected
  arc A28 (-25.7245, 29.1468) -> (-31.1029, 31.7555) centre (-28.8812, 29.4873) ccw projected
  arc A29 (-67.5567, -219.4404) -> (-76.984, -208.5093) centre (-93.2079, -232.032) ccw projected
  arc A30 (-67.5567, -219.4404) -> (-61.8773, -219.482) centre (-64.7066, -218.0413) ccw projected
  line L4 (-61.8773, -219.482) -> (-60.0746, -215.9418) projected
  arc A31 (-60.0746, -215.9418) -> (-60.7584, -212.1608) centre (-62.9039, -214.5011) ccw projected
  arc A32 (-64.7831, -204.3333) -> (-60.7584, -212.1608) centre (-52.1761, -202.7994) ccw projected
  arc A33 (-64.7831, -204.3333) -> (-66.8925, -201.7178) centre (-67.9349, -204.7168) ccw projected
  line L5 (-66.8925, -201.7178) -> (-72.8356, -199.6521) projected
  arc A34 (-72.8356, -199.6521) -> (-76.8242, -201.4676) centre (-73.878, -202.6511) ccw projected
  line L6 (-76.8242, -201.4676) -> (-78.1275, -204.7122) projected
  arc A35 (-78.1275, -204.7122) -> (-76.984, -208.5093) centre (-75.1814, -205.8957) ccw projected
  line L7 (-16.1603, -58.4956) -> (1.0667, -66.5539) projected
  arc A36 (1.0667, -66.5539) -> (4.4026, -66.1514) centre (2.4119, -63.6779) ccw projected
  arc A37 (14.8879, -63.5983) -> (4.4026, -66.1514) centre (12.3652, -76.0452) ccw projected
  arc A38 (14.8879, -63.5983) -> (18.348, -61.9272) centre (15.5186, -60.4865) ccw projected
  line L8 (18.348, -61.9272) -> (26.6735, -45.5766) projected
  arc A39 (26.6735, -45.5766) -> (22.335, -41.3425) centre (23.8442, -44.136) ccw projected
  arc A40 (-11.2736, -45.6176) -> (22.335, -41.3425) centre (0, 0) ccw projected
  arc A41 (-11.2736, -45.6176) -> (-14.9815, -47.5164) centre (-12.0354, -48.6999) ccw projected
  line L9 (-14.9815, -47.5164) -> (-17.7613, -54.4362) projected
  arc A42 (-17.7613, -54.4362) -> (-16.1603, -58.4956) centre (-14.8151, -55.6197) ccw projected
  line L10 (-60.6625, -189.7642) -> (-88.5389, -146.9454) projected
  arc A43 (-88.5389, -146.9454) -> (-92.3649, -145.7242) centre (-91.1997, -148.6777) ccw projected
  arc A44 (-96.1327, -146.5788) -> (-92.3649, -145.7242) centre (-97.0253, -133.9102) ccw projected
  arc A45 (-96.1327, -146.5788) -> (-99.0208, -149.1131) centre (-95.9095, -149.746) ccw projected
  line L11 (-99.0208, -149.1131) -> (-103.0492, -168.9165) projected
  arc A46 (-103.0492, -168.9165) -> (-101.3806, -172.3776) centre (-99.9379, -169.5493) ccw projected
  arc A47 (-94.5445, -182.1568) -> (-101.3806, -172.3776) centre (-107.1516, -183.6907) ccw projected
  arc A48 (-94.5445, -182.1568) -> (-92.4352, -184.7723) centre (-91.3928, -181.7733) ccw projected
  line L12 (-92.4352, -184.7723) -> (-64.3907, -194.5202) projected
  arc A49 (-64.3907, -194.5202) -> (-61.1139, -193.7769) centre (-63.3483, -191.5212) ccw projected
  arc A50 (-61.0938, -193.7571) -> (-61.1139, -193.7769) centre (-52.1761, -202.7994) ccw projected
  arc A51 (-61.0938, -193.7571) -> (-60.6625, -189.7642) centre (-63.3233, -191.4965) ccw projected
  line L13 (-39.1874, -128.4482) -> (-78.3296, -96.1425) projected
  arc A52 (-78.3296, -96.1425) -> (-81.6603, -95.6989) centre (-80.3506, -98.5912) ccw projected
  arc A53 (-86.0064, -96.7983) -> (-81.6603, -95.6989) centre (-86.899, -84.1297) ccw projected
  arc A54 (-86.0064, -96.7983) -> (-88.8946, -99.3326) centre (-85.7833, -99.9655) ccw projected
  line L14 (-88.8946, -99.3326) -> (-92.9229, -119.1359) projected
  arc A55 (-92.9229, -119.1359) -> (-91.2544, -122.5971) centre (-89.8116, -119.7688) ccw projected
  arc A56 (-85.2514, -129.1495) -> (-91.2544, -122.5971) centre (-97.0253, -133.9102) ccw projected
  arc A57 (-85.2514, -129.1495) -> (-82.5342, -131.1262) centre (-82.3079, -127.9593) ccw projected
  line L15 (-82.5342, -131.1262) -> (-51.9243, -133.3141) projected
  arc A58 (-49.8924, -133.4593) -> (-51.9243, -133.3141) centre (-51.8109, -146.0136) ccw projected
  line L16 (-49.8924, -133.4593) -> (-41.4348, -134.0638) projected
  arc A59 (-41.4348, -134.0638) -> (-39.1874, -128.4482) centre (-41.2084, -130.8969) ccw projected
  line L17 (-34.3965, -142.2063) -> (-35.7266, -142.1112) projected
  arc A60 (-35.7266, -142.1112) -> (-39.1245, -145.4252) centre (-35.9529, -145.2781) ccw projected
  arc A61 (-46.8252, -157.694) -> (-39.1245, -145.4252) centre (-51.8109, -146.0136) ccw projected
  line L18 (-46.8252, -157.694) -> (-63.3439, -164.7448) projected
  arc A62 (-63.3886, -164.7638) -> (-63.3439, -164.7448) centre (-68.3295, -153.0643) ccw projected
  arc A63 (-63.3886, -164.7638) -> (-64.8141, -169.4209) centre (-62.1533, -167.6886) ccw projected
  line L19 (-64.8141, -169.4209) -> (-52.1408, -188.8873) projected
  arc A64 (-52.1408, -188.8873) -> (-50.0192, -190.2839) centre (-49.48, -187.1551) ccw projected
  arc A65 (-49.6538, -190.3524) -> (-50.0192, -190.2839) centre (-52.1761, -202.7994) ccw projected
  arc A66 (-49.6538, -190.3524) -> (-46.1939, -188.6813) centre (-49.0232, -187.2407) ccw projected
  line L20 (-46.1939, -188.6813) -> (-27.8038, -152.5648) projected
  arc A67 (-27.8038, -152.5648) -> (-28.4876, -148.7838) centre (-30.6331, -151.1242) ccw projected
  arc A68 (-31.6794, -144.183) -> (-28.4876, -148.7838) centre (-19.9055, -139.4223) ccw projected
  arc A69 (-31.6794, -144.183) -> (-34.3965, -142.2063) centre (-34.6229, -145.3732) ccw projected
  circle A70 centre (-19.9055, -139.4223) radius 5.588 projected
  circle A71 centre (12.3652, -76.0452) radius 5.588 projected
  circle A72 centre (-52.1761, -202.7994) radius 5.588 projected
  circle A73 centre (-10.4425, -25.9152) radius 6.731 projected
  circle A74 centre (-6.7844, 27.1038) radius 6.731 projected
  line L21 (-56.4266, -250.7606) -> (56.5866, -28.8133) projected
  arc A75 (-133.6545, -223.8044) -> (-56.4266, -250.7606) centre (-93.2079, -232.032) ccw projected
  line L22 (-94.387, -30.7661) -> (-133.6545, -223.8044) projected
  arc A76 (-79.8174, 0.8878) -> (-94.387, -30.7661) centre (-19.7163, -45.9555) ccw projected
  line L23 (-50.0843, 39.0361) -> (-79.8174, 0.8878) projected
  arc A77 (56.5866, -28.8133) -> (-50.0843, 39.0361) centre (0, 0) ccw projected
  circle A78 centre (0, 0) radius 13.4938 projected
  line L24 (-92.6287, -239.1078) -> (-87.8947, -227.3231) projected
  arc A79 (-87.8947, -227.3231) -> (-93.7871, -224.9561) centre (-90.8409, -226.1396) ccw projected
  line L25 (-93.7871, -224.9561) -> (-98.521, -236.7409) projected
  arc A80 (-98.521, -236.7409) -> (-92.6287, -239.1078) centre (-95.5749, -237.9244) ccw projected
  circle A81 centre (23.6807, 14.8279) radius 6.731 projected
  circle A82 centre (-27.8737, 1.9232) radius 6.731 projected
  circle A83 centre (21.4199, -17.9397) radius 6.731 projected
  line L26 (-85.1984, -201.8718) -> (-84.1423, -199.2428) projected
  arc A84 (-84.1423, -199.2428) -> (-86.0461, -195.0603) centre (-87.0885, -198.0593) ccw projected
  line L27 (-86.0461, -195.0603) -> (-94.937, -191.9699) projected
  arc A85 (-94.937, -191.9699) -> (-98.2138, -192.7133) centre (-95.9794, -194.9689) ccw projected
  arc A86 (-106.259, -196.3593) -> (-98.2138, -192.7133) centre (-107.1516, -183.6907) ccw projected
  arc A87 (-106.259, -196.3593) -> (-109.1471, -198.8936) centre (-106.0358, -199.5265) ccw projected
  line L28 (-109.1471, -198.8936) -> (-109.9237, -202.7115) projected
  arc A88 (-109.9237, -202.7115) -> (-105.452, -206.2132) centre (-106.8124, -203.3444) ccw projected
  arc A89 (-88.6509, -203.8227) -> (-105.452, -206.2132) centre (-93.2079, -232.032) ccw projected
  arc A90 (-88.6509, -203.8227) -> (-85.1984, -201.8718) centre (-88.1445, -200.6883) ccw projected
  line L29 (-24.5425, -50.8749) -> (-22.0524, -44.676) projected
  arc A91 (-22.0524, -44.676) -> (-23.4164, -40.7398) centre (-24.9986, -43.4925) ccw projected
  arc A92 (-46.9122, 2.703) -> (-23.4164, -40.7398) centre (0, 0) ccw projected
  arc A93 (-46.9122, 2.703) -> (-52.5861, 4.8375) centre (-50.0819, 2.8857) ccw projected
  line L30 (-52.5861, 4.8375) -> (-64.7921, -10.8231) projected
  arc A94 (-64.7921, -10.8231) -> (-70.5556, -19.8503) centre (-19.7163, -45.9555) ccw projected
  arc A95 (-70.5556, -19.8503) -> (-69.5395, -23.9103) centre (-67.7312, -21.3006) ccw projected
  arc A96 (-64.0748, -34.1198) -> (-69.5395, -23.9103) centre (-76.7728, -34.3492) ccw projected
  arc A97 (-64.0748, -34.1198) -> (-62.2456, -36.9383) centre (-60.9004, -34.0624) ccw projected
  line L31 (-62.2456, -36.9383) -> (-28.8339, -52.5673) projected
  arc A98 (-28.8339, -52.5673) -> (-24.5425, -50.8749) centre (-27.4887, -49.6914) ccw projected
  arc A99 (-75.8802, -47.0178) -> (-68.8102, -44.243) centre (-76.7728, -34.3492) ccw projected
  arc A100 (-75.8802, -47.0178) -> (-78.7683, -49.5521) centre (-75.657, -50.185) ccw projected
  line L32 (-78.7683, -49.5521) -> (-82.7967, -69.3554) projected
  arc A101 (-82.7967, -69.3554) -> (-81.1281, -72.8166) centre (-79.6854, -69.9883) ccw projected
  arc A102 (-75.9857, -77.6344) -> (-81.1281, -72.8166) centre (-86.899, -84.1297) ccw projected
  arc A103 (-75.9857, -77.6344) -> (-72.9996, -79.1751) centre (-73.2574, -76.0105) ccw projected
  line L33 (-72.9996, -79.1751) -> (-14.1782, -74.3844) projected
  arc A104 (-14.1782, -74.3844) -> (-13.0907, -68.3439) centre (-14.436, -71.2199) ccw projected
  line L34 (-13.0907, -68.3439) -> (-65.4743, -43.8405) projected
  arc A105 (-65.4743, -43.8405) -> (-68.8102, -44.243) centre (-66.8195, -46.7164) ccw projected
  arc A106 (-17.3829, -126.9753) -> (-25.1442, -127.8531) centre (-19.9055, -139.4223) ccw projected
  arc A107 (-17.3829, -126.9753) -> (-13.923, -125.3043) centre (-16.7523, -123.8636) ccw projected
  line L35 (-13.923, -125.3043) -> (4.4671, -89.1879) projected
  arc A108 (4.4671, -89.1879) -> (3.7832, -85.4068) centre (1.6378, -87.7473) ccw projected
  arc A109 (1.4518, -82.5405) -> (3.7832, -85.4068) centre (12.3652, -76.0452) ccw projected
  arc A110 (1.4518, -82.5405) -> (-1.5342, -80.9998) centre (-1.2765, -84.1643) ccw projected
  line L36 (-1.5342, -80.9998) -> (-69.4404, -86.5304) projected
  arc A111 (-69.4404, -86.5304) -> (-71.2037, -92.1436) centre (-69.1827, -89.6949) ccw projected
  line L37 (-71.2037, -92.1436) -> (-28.4749, -127.4095) projected
  arc A112 (-28.4749, -127.4095) -> (-25.1442, -127.8531) centre (-26.4539, -124.9608) ccw projected
  circle A113 centre (-68.3295, -153.0643) radius 6.731 projected
  circle A114 centre (-51.8109, -146.0136) radius 6.731 projected
  circle A115 centre (-56.5448, -157.7983) radius 3.175 projected
  circle A116 centre (-56.5448, -157.7983) radius 12.7
  line L38 (-38.1697, -143.0052) -> (-47.599, -148.7837)
  point P0 (0, 0)
  point P1 (-43.972, -156.0056)
  point P2 (-65.2604, -167.0356)
  dimension "d61" = 25.4
  constraints: 2 end point, 1 coincident, 1 point on circle, 3 other
extrude "Extrusion14" cut sketch "Sketch14" against normal blind 6.35 contours A5 A4 A3 A2 L1 A1 L0 A0 | A10 A9 A8 A7 L2 A6 | A11 A16 A15 A14 A13 A12 | A17 A22 A21 A20 A19 A18 | A28 A27 A26 A25 A24 L3 A23 | A69 A68 A67 L20 A66 A65 A64 L19 A63 A116 A61 A60 L17 | A60 A61 A116 A114 L38 | A114 A116 L38 picked at (-46.0957, -148.1343)
fillet "Fillet4" radius 3.175 1 edges at (-65.2604, -167.0356, 3.175)
fillet "Fillet5" radius 3.175 2 edges at (-47.599, -148.7837, 3.175) (-38.1697, -143.0052, 3.175)
body "Solid1"
